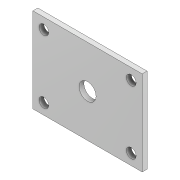
# Autodesk Inventor part: Soporta Potenciómetro
Saved by Autodesk Inventor 2020 (Build 240168000, 168)
## iProperties
Created: 2020-09-22
Part Number: Soporta Potenciómetro
Material: Aluminum 1100-H14
Document SubType Name: Modeling
Designer: Hernan
Density: 2.7 g/cm^3
Appearance: Satin
Author: Hernan
Autodesk Inventor part; units mm, degrees
ref_plane "YZ Plane" through (0, 0, 0) normal (1, 0, 0) x (0, 1, 0)
ref_plane "XZ Plane" through (0, 0, 0) normal (0, 1, 0) x (-1, 0, 0)
ref_plane "XY Plane" through (0, 0, 0) normal (0, 0, 1) x (1, 0, 0)
sketch "Sketch1" plane through (0, 0, 0) normal (0, 0, 1) x (1, 0, 0)
  line L0 (-16.8673, 67.8112) -> (-16.8673, 32.8112)
  line L1 (-16.8673, 32.8112) -> (-61.8673, 32.8112)
  line L2 (-61.8673, 32.8112) -> (-61.8673, 67.8112)
  line L3 (-61.8673, 67.8112) -> (-16.8673, 67.8112)
  circle A0 centre (-57.3673, 37.3112) radius 2
  circle A1 centre (-21.3673, 37.3112) radius 2
  circle A2 centre (-21.3673, 63.3112) radius 2
  circle A3 centre (-57.3673, 63.3112) radius 2
  circle A4 centre (-39.3673, 50.3112) radius 3.5
  point P0 (0, 0)
  dimension "d35" = 35
  dimension "d36" = 35
  dimension "d37" = 45
  dimension "d38" = 45
  dimension "d39" = 7
  dimension "d40" = 13
  dimension "d41" = 4
  dimension "d42" = 13
  dimension "d43" = 13
  dimension "d44" = 13
  dimension "d45" = 4
  dimension "d46" = 4
  dimension "d47" = 4
  dimension "d48" = 18
  dimension "d49" = 17.5
  dimension "d50" = 22.5
  dimension "d51" = 18
  dimension "d52" = 18
  dimension "d53" = 18
  constraints: 8 end point, 5 centre point, 1 parallel, 1 perpendicular
  measures "d35" distance of L0.start L0.end
  measures "d36" distance of L1.end L2.end
  measures "d37" distance of L0.end L1.end
  measures "d38" distance of L2.end L0.start
  measures "d39" diameter of A4
  measures "d40" vertical distance of A2.centre A4.centre
  measures "d41" diameter of A2
  measures "d42" vertical distance of A1.centre A4.centre
  measures "d43" vertical distance of A3.centre A4.centre
  measures "d44" vertical distance of A0.centre A4.centre
  measures "d45" diameter of A3
  measures "d46" diameter of A1
  measures "d47" diameter of A0
  measures "d48" horizontal distance of A3.centre A4.centre
  measures "d49" distance from line of L1 A4.centre
  measures "d50" distance from line of L0 A4.centre
  measures "d51" horizontal distance of A0.centre A4.centre
  measures "d52" horizontal distance of A4.centre A2.centre
  measures "d53" horizontal distance of A4.centre A1.centre
extrude "Extrusion1" add sketch "Sketch1" along normal blind 2
equation "\"d36\" = d35"
equation "\"d38\" = d37"
equation "\"d42\" = d40"
equation "\"d43\" = d40"
equation "\"d44\" = d42"
equation "\"d45\" = d41"
equation "\"d46\" = d41"
equation "\"d47\" = d46"
equation "\"d51\" = d48"
equation "\"d52\" = d48"
equation "\"d53\" = d51"
body "Solid1"
